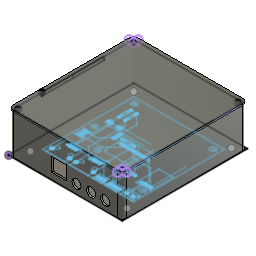
krabice - štít v2 (Autodesk Fusion 360 design; units mm, degrees)
Autodesk Fusion 360 part; units mm, degrees
note: some values were not read from the file. Set by a fixed rule: which sketch regions a step uses.
sketch "Base" plane through (0, 0, 0) normal (0, 1, 0) x (1, 0, 0) in component "Top"
  line L0 (0, 0) -> (100, 0)
  line L1 (100, 0) -> (100, 110)
  line L2 (100, 110) -> (0, 110)
  line L3 (0, 110) -> (0, 0)
  dimension "d6" = 100
  dimension "d7" = 110
  constraint horizontal L0
  constraint vertical L1
  constraint horizontal L2
  constraint vertical L3
  constraint coincident L0.start L3.end
  measures "d6" distance of L0.start L0.end
  measures "d7" distance of L0.start L2.end
extrude "Extrude1" add sketch "Base" along normal blind 35 makes body 1 in component "Top"
fillet "Fillet1" radius 4 4 edges at (100, 17.5, 0) (0, 17.5, 0) (100, 17.5, -110) (0, 17.5, -110) on bodies 1 in component "Top"
shell "Shell1" thickness 1.5 removed faces 1 at (33.3333, 35, -72) on bodies 1 in component "Top"
sketch "Knob" plane through (1.5, 0, 0) normal (1, 0, 0) x (0, 0, -1) in component "Top"
  line L0 (106, 1.5) -> (106, 35)
  line L1 (106, 35) -> (4, 35)
  line L2 (4, 35) -> (4, 1.5)
  line L3 (4, 1.5) -> (106, 1.5)
  line L4 (27.5, 35) -> (82.5, 35)
  line L5 (82.5, 35) -> (82.5, 32)
  line L6 (82.5, 32) -> (27.5, 32)
  line L7 (27.5, 32) -> (27.5, 35)
  line L8 (55, 35) -> (55, 32) construction
  dimension "d12" = 55
  dimension "d13" = 3
  constraint horizontal L4
  constraint vertical L5
  constraint horizontal L6
  constraint vertical L7
  constraint coincident L1 L4.start
  constraint midpoint L1 L8.start
  constraint midpoint L6 L8.end
  constraint vertical L8
  measures "d12" distance of L5.end L6.end
  measures "d13" distance of L4.end L5.end
extrude "Extrude2" add sketch "Knob" along normal blind 6 draft -45 contours L1 L4 L5 L6 L7 bodies 1 in component "Top"
ref_plane "WorkPlane2" through (50, 17.5, -55) normal (-1, 0, 0) x (0, 0, 1) in component "Top"
mirror "Mirror1" about plane through (50, 17.5, -55) normal (-1, 0, 0) of "Extrude2" in component "Top"
sketch "Top" plane through (0, 35, 0) normal (0, 1, 0) x (-1, 0, 0) in component "Base"
  line L0 (-100, -4) -> (-100, -106)
  arc A0 (-100, -106) -> (-96, -110) centre (-96, -106) ccw
  line L1 (-96, -110) -> (-4, -110)
  arc A1 (-4, -110) -> (0, -106) centre (-4, -106) ccw
  line L2 (0, -106) -> (0, -4)
  arc A2 (0, -4) -> (-4, 0) centre (-4, -4) ccw
  line L3 (-4, 0) -> (-96, 0)
  arc A3 (-96, 0) -> (-100, -4) centre (-96, -4) ccw
  arc A4 (-96, -1.5) -> (-98.5, -4) centre (-96, -4) ccw
  line L4 (-96, -1.5) -> (-4, -1.5)
  arc A5 (-1.5, -4) -> (-4, -1.5) centre (-4, -4) ccw
  line L5 (-1.5, -27.5) -> (-1.5, -82.5)
  arc A6 (-4, -108.5) -> (-1.5, -106) centre (-4, -106) ccw
  line L6 (-4, -108.5) -> (-96, -108.5)
  arc A7 (-98.5, -106) -> (-96, -108.5) centre (-96, -106) ccw
  line L7 (-98.5, -82.5) -> (-98.5, -27.5)
  line L8 (-98.5, -27.5) -> (-98.5, -4)
  line L9 (-1.5, -4) -> (-1.5, -27.5)
  line L10 (-1.5, -82.5) -> (-1.5, -106)
  line L11 (-98.5, -106) -> (-98.5, -82.5)
extrude "Extrude1'" add sketch "Top" along normal blind 1.5 separate body contours L0 A0 L1 A1 L2 A2 L3 A3 | A4 L4 A5 L5 A6 L6 A7 L7 L8 L9 L10 L11 makes body 2 in component "Base"
sketch "Lip" plane through (0, 35, 0) normal (0, -1, 0) x (1, 0, 0) in component "Base"
  arc A0 (100, -4) -> (96, 0) centre (96, -4) ccw
  line L0 (96, 0) -> (4, 0)
  arc A1 (4, 0) -> (0, -4) centre (4, -4) ccw
  line L1 (0, -4) -> (0, -106)
  arc A2 (0, -106) -> (4, -110) centre (4, -106) ccw
  line L2 (4, -110) -> (96, -110)
  arc A3 (96, -110) -> (100, -106) centre (96, -106) ccw
  line L3 (100, -106) -> (100, -4)
  line L4 (98.3, -106) -> (98.3, -4)
  arc A4 (98.3, -4) -> (96, -1.7) centre (96, -4) ccw
  line L5 (96, -1.7) -> (4, -1.7)
  arc A5 (4, -1.7) -> (1.7, -4) centre (4, -4) ccw
  line L6 (1.7, -4) -> (1.7, -106)
  arc A6 (1.7, -106) -> (4, -108.3) centre (4, -106) ccw
  line L7 (4, -108.3) -> (96, -108.3)
  arc A7 (96, -108.3) -> (98.3, -106) centre (96, -106) ccw
  dimension "d19" = 1.7
extrude "Extrude2'" add sketch "Lip" along normal blind 3 contours L4 A4 L5 A5 L6 A6 L7 A7 bodies 2 in component "Base"
extrude "Extrude3" cut sketch "Knob" along normal blind 3 draft -45 from surface at 0.2 contours L1 L4 L5 L6 L7 bodies 2 in component "Base"
mirror "Mirror1'" about plane through (50, 17.5, -55) normal (-1, 0, 0) of "Extrude3" in component "Base"
shell "Shell1'" thickness 1.5 removed faces 1 at (66.1, 32, -64.1667) on bodies 2 in component "Base"
chamfer "Chamfer1" distance 0.6 angle 45 2 edges at (1.7, 32, -55) (98.3, 32, -55) on bodies 2 in component "Base"
sketch "PCB Mount" plane through (0, 35, 0) normal (0, -1, 0) x (1, 0, 0) in component "Base"
  arc A0 (100, -4) -> (96, 0) centre (96, -4) ccw construction
  arc A1 (0, -106) -> (4, -110) centre (4, -106) ccw construction
sketch "PCB_Slave_2021-08-24" plane through (0, 1.5, -25) normal (0, 1, 0) x (1, 0, 0)
  line L0 (57.578, 9.4539) -> (57.578, 31.463)
  line L1 (85.899, 11.27) -> (84.5401, 12.6289)
  line L2 (84.5401, 12.6289) -> (82.7926, 12.6289)
  line L3 (30.3848, 47.0992) -> (30.3848, 43.147)
  line L4 (34.6494, 52.9946) -> (34.6494, 38.194)
  line L5 (51.482, 37.559) -> (57.578, 31.463)
  line L6 (49.958, 35.4) -> (49.958, 31.463)
  line L7 (43.9915, 8.4836) -> (50.245, 8.4836)
  line L8 (30.3848, 14.9276) -> (39.6304, 5.682)
  line L9 (20.875, 44.4018) -> (21.9215, 44.4018)
  line L10 (21.9215, 44.4018) -> (22.968, 43.3553)
  line L11 (62.465, -3.7363) -> (64.0169, -5.2857)
  line L12 (88.439, 42.131) -> (88.439, 11.27)
  line L13 (21.698, 9.1212) -> (21.698, 18.697)
  line L14 (30.3848, 43.147) -> (30.3848, 14.9276)
  line L15 (26.082, 61.562) -> (34.6494, 52.9946)
  line L16 (72.437, 13.683) -> (65.198, 20.922)
  line L17 (26.082, 51.402) -> (30.3848, 47.0992)
  line L18 (60.118, 9.4539) -> (73.3057, -3.7363)
  line L19 (64.0169, -5.2857) -> (74.2963, -5.2857)
  line L20 (65.198, 20.922) -> (65.198, 31.463)
  line L21 (70.7657, -3.7363) -> (57.578, 9.4539)
  line L22 (74.2963, -5.2857) -> (75.8457, -3.7363)
  line L23 (61.5582, 14.4018) -> (62.277, 13.683)
  line L24 (60.118, 31.463) -> (60.118, 9.4539)
  line L25 (59.102, 32.479) -> (60.118, 31.463)
  line L26 (39.6304, 5.682) -> (43.7299, 5.682)
  line L27 (43.7299, 5.682) -> (45.2615, 7.2136)
  line L28 (87.6364, -3.335) -> (83.359, 0.9424)
  line L29 (20.875, 51.402) -> (20.875, 44.4018)
  line L30 (82.0687, -2.7686) -> (82.6376, -3.335)
  line L31 (22.968, 43.3553) -> (22.968, 9.7536)
  line L32 (66.8033, 35.6083) -> (64.8373, 33.6423)
  line L33 (64.8373, 33.6423) -> (82.7926, 15.6871)
  line L34 (61.5582, 41.0718) -> (61.5582, 14.4018)
  line L35 (17.3139, 23.081) -> (21.6218, 27.3888)
  line L36 (50.245, 8.4836) -> (62.465, -3.7363)
  line L37 (24.238, 7.2136) -> (23.603, 7.2136)
  line L38 (83.359, 0.9424) -> (83.359, 11.27)
  line L39 (43.9915, 8.4836) -> (42.7215, 7.2136)
  line L40 (49.958, 13.1801) -> (49.958, 31.463)
  line L41 (23.603, 7.2136) -> (21.698, 9.1212)
  line L42 (82.7926, 15.6871) -> (82.7926, 12.6289)
  line L43 (43.9915, 9.7536) -> (43.9915, 8.4836)
  line L44 (82.7926, 12.6289) -> (82.0687, 11.905)
  line L45 (64.8373, 33.6423) -> (62.658, 31.463)
  line L46 (21.6218, 27.3888) -> (21.6218, 43.147)
  line L47 (21.698, 18.697) -> (17.3139, 23.081)
  line L48 (49.704, 35.654) -> (49.958, 35.4)
  line L49 (46.5315, 9.7536) -> (49.958, 13.1801)
  line L50 (20.875, 44.4018) -> (19.6202, 43.147)
  line L51 (82.0687, 11.905) -> (82.0687, -2.7686)
  line L52 (92, 73) -> (92, -7)
  line L53 (12, 73) -> (92, 73)
  line L54 (12, -7) -> (12, 73)
  line L55 (92, -7) -> (12, -7)
  line L56 (66.6763, -5.2857) -> (68.2257, -3.7363)
  line L57 (57.385, -3.7363) -> (58.9369, -5.2857)
  line L58 (36.496, 20.541) -> (17.3139, 20.541)
  line L59 (65.198, 38.194) -> (34.6494, 38.194)
  line L60 (41.5227, 8.415) -> (25.4394, 8.415)
  line L61 (68.2257, 9.4717) -> (72.437, 13.683)
  line L62 (53.768, 31.0007) -> (53.768, 32.0472)
  line L63 (73.707, 26.002) -> (58.7667, 26.002)
  line L64 (42.7215, 7.2136) -> (41.5227, 8.415)
  line L65 (82.6376, -3.335) -> (76.247, -3.335)
  line L66 (47.418, 31.463) -> (36.496, 20.541)
  line L67 (52.7012, 33.114) -> (34.6494, 33.114)
  line L68 (22.5412, 40.226) -> (19.6202, 43.147)
  line L69 (26.082, 61.562) -> (20.875, 61.562)
  line L70 (31.4008, 44.163) -> (30.3848, 43.147)
  line L71 (65.198, 42.004) -> (65.198, 38.194)
  line L72 (76.247, -3.335) -> (75.8457, -3.7363)
  line L73 (58.7667, 26.002) -> (53.768, 31.0007)
  line L74 (88.439, 11.27) -> (73.707, 26.002)
  line L75 (59.925, -3.7363) -> (62.277, -1.3843)
  line L76 (68.2257, -3.7363) -> (68.2257, 9.4717)
  line L77 (25.4394, 8.415) -> (24.238, 7.2136)
  line L78 (55.927, 44.163) -> (31.4008, 44.163)
  line L79 (17.3139, 25.621) -> (27.1564, 25.621)
  line L80 (62.277, -1.3843) -> (62.277, 13.683)
  line L81 (39.544, 35.654) -> (34.6494, 35.654)
  line L82 (53.26, 40.226) -> (22.5412, 40.226)
  line L83 (28.3832, 43.147) -> (21.6218, 43.147)
  line L84 (27.1564, 25.621) -> (34.6494, 33.114)
  line L85 (65.198, 38.194) -> (65.198, 31.463)
  line L86 (58.9369, -5.2857) -> (66.6763, -5.2857)
  line L87 (53.768, 32.0472) -> (52.7012, 33.114)
  line L88 (64.817, 14.699) -> (69.897, 14.699)
  line L89 (63.9349, -0.735) -> (63.9349, -7.035)
  line L90 (55.9149, -0.735) -> (55.9149, -7.035)
  line L91 (55.9149, -7.035) -> (63.9349, -7.035)
  line L92 (33.3794, 31.844) -> (33.3794, 39.464)
  line L93 (55.9149, -0.735) -> (63.9349, -0.735)
  line L94 (33.3794, 39.464) -> (35.9194, 39.464)
  line L95 (64.817, 12.667) -> (64.817, 14.699)
  line L96 (66.756, -0.735) -> (77.316, -0.735)
  line L97 (30.384, 41.147) -> (30.384, 42.163)
  line L98 (69.897, 13.683) -> (72.437, 13.683)
  line L99 (35.9194, 39.464) -> (35.9194, 31.844)
  line L100 (20.3141, 27.091) -> (14.0141, 27.091)
  line L101 (66.756, -0.735) -> (66.756, -7.035)
  line L102 (66.756, -2.277) -> (77.316, -2.277)
  line L103 (55.9149, -2.277) -> (63.9349, -2.277)
  line L104 (20.3141, 27.091) -> (20.3141, 19.071)
  line L105 (15.7524, 27.091) -> (15.7524, 19.071)
  line L106 (66.756, -6.5047) -> (77.316, -6.5047)
  line L107 (78.2789, 21.43) -> (78.2789, 29.05)
  line L108 (79.5489, 10.3708) -> (79.5489, 10)
  line L109 (65.7314, 18.7376) -> (41.83, 18.763)
  line L110 (62.277, 13.683) -> (64.817, 13.683)
  line L111 (19.1049, 44.6469) -> (20.1209, 44.6469)
  line L112 (79.5489, 10) -> (89.7089, 10)
  line L113 (20.3141, 19.071) -> (14.0141, 19.071)
  line L114 (66.756, -5.2967) -> (77.316, -5.2967)
  line L115 (79.5489, 12.54) -> (79.5489, 10.3708)
  line L116 (69.897, 14.699) -> (69.897, 12.667)
  line L117 (39.798, 20.7188) -> (39.798, 30.701)
  line L118 (14.0141, 27.091) -> (14.0141, 19.071)
  line L119 (21.891, 53.942) -> (19.859, 53.942)
  line L120 (19.859, 53.942) -> (19.859, 59.022)
  line L121 (69.897, 12.667) -> (64.817, 12.667)
  line L122 (41.83, 32.733) -> (65.7314, 32.733)
  line L123 (66.756, -7.035) -> (77.316, -7.035)
  line L124 (90.8519, 29.05) -> (90.8519, 8.73)
  line L125 (19.621, 45.147) -> (19.621, 44.131)
  line L126 (19.859, 59.022) -> (21.891, 59.022)
  line L127 (27.098, 59.022) -> (27.098, 53.942)
  line L128 (55.9149, -5.2967) -> (63.9349, -5.2967)
  line L129 (25.066, 59.022) -> (27.098, 59.022)
  line L130 (42.084, 36.67) -> (47.164, 36.67)
  line L131 (47.164, 35.654) -> (49.704, 35.654)
  line L132 (80.137, 0.665) -> (90.137, 0.665)
  line L133 (47.164, 36.67) -> (47.164, 34.638)
  line L134 (80.137, 0.665) -> (80.137, -7.035)
  line L135 (35.9194, 31.844) -> (33.3794, 31.844)
  line L136 (89.7089, 12.54) -> (79.5489, 12.54)
  line L137 (20.875, 53.942) -> (20.875, 51.402)
  line L138 (55.9149, -6.5047) -> (63.9349, -6.5047)
  line L139 (78.2789, 8.73) -> (78.2789, 21.43)
  line L140 (30.9001, 41.6471) -> (29.8841, 41.6471)
  line L141 (26.082, 53.942) -> (26.082, 51.402)
  line L142 (27.098, 53.942) -> (25.066, 53.942)
  line L143 (47.164, 34.638) -> (42.084, 34.638)
  line L144 (18.772, 27.091) -> (18.772, 19.071)
  line L145 (77.316, -0.735) -> (77.316, -7.035)
  line L146 (67.738, 30.7264) -> (67.738, 20.7442)
  line L147 (25.066, 53.942) -> (25.066, 59.022)
  line L148 (90.8519, 8.73) -> (78.2789, 8.73)
  line L149 (90.137, 0.665) -> (90.137, -7.035)
  line L150 (42.084, 34.638) -> (42.084, 36.67)
  line L151 (80.137, -7.035) -> (90.137, -7.035)
  line L152 (20.875, 61.562) -> (20.875, 59.022)
  line L153 (21.891, 59.022) -> (21.891, 53.942)
  line L154 (14.5444, 27.091) -> (14.5444, 19.071)
  line L155 (39.544, 35.654) -> (42.084, 35.654)
  line L156 (26.082, 61.562) -> (26.082, 59.022)
  line L157 (89.7089, 10) -> (89.7089, 12.54)
  line L158 (78.2789, 29.05) -> (90.8519, 29.05)
  line L159 (36.0522, 11.365) -> (51.9323, 11.365)
  arc A0 (65.739, 18.733) -> (67.738, 20.733) centre (65.739, 20.732) ccw
  line L160 (51.9323, -7.035) -> (36.0522, -7.035)
  arc A1 (39.83, 20.763) -> (41.829, 18.763) centre (41.829, 20.762) ccw
  line L161 (90.845, -1.7086) -> (90.217, -1.7086)
  arc A2 (67.738, 30.733) -> (65.739, 32.733) centre (65.739, 30.734) ccw
  line L162 (15.0279, 11.365) -> (30.908, 11.365)
  line L163 (80.137, -5.1796) -> (90.137, -5.1796)
  circle A3 centre (20.621, 43.147) radius 2.5001
  line L164 (80.137, -1.1344) -> (90.137, -1.1344)
  line L165 (30.908, 11.365) -> (30.908, -7.035)
  line L166 (51.9323, 11.365) -> (51.9323, -7.035)
  line L167 (36.0522, -7.035) -> (36.0522, 11.365)
  line L168 (30.908, -7.035) -> (15.0279, -7.035)
  line L169 (15.0279, -7.035) -> (15.0279, 11.365)
  circle A4 centre (29.384, 43.147) radius 2.5001
  arc A5 (41.797, 32.701) -> (39.798, 30.701) centre (41.797, 30.702) ccw
  line L170 (90.845, -0.668) -> (90.845, -1.7086)
  line L171 (90.217, -0.668) -> (90.845, -0.668)
  line L172 (69.897, 13.683) -> (72.437, 13.683)
  line L173 (42.084, 34.638) -> (42.084, 36.67)
  line L174 (64.817, 12.667) -> (64.817, 14.699)
  line L175 (27.098, 59.022) -> (27.098, 53.942)
  line L176 (20.875, 61.562) -> (20.875, 59.022)
  line L177 (25.066, 53.942) -> (25.066, 59.022)
  line L178 (47.164, 36.67) -> (47.164, 34.638)
  line L179 (26.082, 53.942) -> (26.082, 51.402)
  line L180 (27.098, 53.942) -> (25.066, 53.942)
  line L181 (69.897, 12.667) -> (64.817, 12.667)
  line L182 (21.891, 59.022) -> (21.891, 53.942)
  line L183 (42.084, 36.67) -> (47.164, 36.67)
  line L184 (21.891, 53.942) -> (19.859, 53.942)
  line L185 (39.544, 35.654) -> (42.084, 35.654)
  line L186 (69.897, 14.699) -> (69.897, 12.667)
  line L187 (19.859, 53.942) -> (19.859, 59.022)
  line L188 (47.164, 35.654) -> (49.704, 35.654)
  line L189 (26.082, 61.562) -> (26.082, 59.022)
  line L190 (62.277, 13.683) -> (64.817, 13.683)
  line L191 (25.066, 59.022) -> (27.098, 59.022)
  line L192 (47.164, 34.638) -> (42.084, 34.638)
  line L193 (19.859, 59.022) -> (21.891, 59.022)
  line L194 (20.875, 53.942) -> (20.875, 51.402)
  line L195 (64.817, 14.699) -> (69.897, 14.699)
  circle A6 centre (47.8023, 7.2149) radius 0.8008
  circle A7 centre (15.2179, -2.1399) radius 1.3008
  circle A8 centre (42.7223, 7.215) radius 0.4805
  circle A9 centre (51.7423, -2.14) radius 0.8325
  circle A10 centre (46.5323, 9.755) radius 0.4805
  circle A11 centre (41.4523, 9.755) radius 0.4805
  circle A12 centre (45.2623, 7.215) radius 0.4805
  circle A13 centre (87.6371, -3.335) radius 1.1254
  circle A14 centre (51.7423, -2.1399) radius 1.3008
  circle A15 centre (28.048, 9.755) radius 0.4805
  circle A16 centre (41.4523, 9.7549) radius 0.8008
  circle A17 centre (42.7223, 7.2149) radius 0.8008
  circle A18 centre (22.968, 9.755) radius 0.4805
  circle A19 centre (46.5323, 9.7549) radius 0.8008
  circle A20 centre (20.428, 9.7549) radius 0.8008
  circle A21 centre (49.0723, 9.755) radius 0.4805
  circle A22 centre (36.2423, -2.14) radius 0.8325
  circle A23 centre (43.9923, 9.755) radius 0.4805
  circle A24 centre (22.968, 9.7549) radius 0.8008
  circle A25 centre (28.048, 9.7549) radius 0.8008
  circle A26 centre (15.218, -2.14) radius 0.8325
  circle A27 centre (80.819, 11.27) radius 0.5317
  circle A28 centre (82.637, -3.335) radius 0.7162
  circle A29 centre (45.2623, 7.2149) radius 0.8008
  circle A30 centre (25.508, 9.755) radius 0.4805
  circle A31 centre (36.2423, -2.1399) radius 1.3008
  circle A32 centre (47.8023, 7.215) radius 0.4805
  circle A33 centre (43.9923, 9.7549) radius 0.8008
  circle A34 centre (40.1823, 7.2149) radius 0.4805
  circle A35 centre (19.158, 7.2149) radius 0.4805
  circle A36 centre (25.508, 9.7549) radius 0.8008
  circle A37 centre (49.0723, 9.7549) radius 0.8008
  circle A38 centre (24.238, 7.215) radius 0.4805
  circle A39 centre (34.6494, 38.194) radius 0.9008
  circle A40 centre (34.6494, 33.114) radius 0.9008
  circle A41 centre (34.6494, 35.654) radius 0.9008
  circle A42 centre (57.578, 31.463) radius 0.4877
  circle A43 centre (57.578, 31.463) radius 0.8128
  circle A44 centre (65.198, 31.463) radius 0.4877
  circle A45 centre (17.3141, 20.541) radius 0.6665
  circle A46 centre (65.198, 31.463) radius 0.8128
  circle A47 centre (17.3142, 25.621) radius 1.0254
  circle A48 centre (17.3141, 25.621) radius 0.6665
  circle A49 centre (62.658, 31.463) radius 0.4877
  circle A50 centre (34.6494, 33.114) radius 0.5829
  circle A51 centre (34.6494, 38.194) radius 0.5829
  circle A52 centre (34.6494, 35.654) radius 0.5829
  circle A53 centre (73.3059, -3.7351) radius 1.0254
  circle A54 centre (68.2259, -3.7351) radius 1.0254
  circle A55 centre (20.875, 61.562) radius 0.4875
  circle A56 centre (44.878, 31.463) radius 0.4877
  circle A57 centre (21.621, 43.147) radius 0.4156
  circle A58 centre (55.038, 31.463) radius 0.4877
  circle A59 centre (17.3142, 23.081) radius 1.0254
  circle A60 centre (62.277, 13.683) radius 0.8128
  circle A61 centre (52.498, 31.463) radius 0.4877
  circle A62 centre (62.658, 31.463) radius 0.8128
  circle A63 centre (59.925, -3.7351) radius 1.0254
  circle A64 centre (57.3849, -3.735) radius 0.6665
  circle A65 centre (85.899, 11.27) radius 0.8508
  circle A66 centre (83.359, 11.27) radius 0.8508
  circle A67 centre (17.3142, 20.541) radius 1.0254
  circle A68 centre (19.621, 43.147) radius 0.6754
  circle A69 centre (55.038, 31.463) radius 0.8128
  circle A70 centre (72.437, 13.683) radius 0.8128
  circle A71 centre (59.9249, -3.735) radius 0.6665
  circle A72 centre (57.385, -3.7351) radius 1.0254
  circle A73 centre (21.621, 43.147) radius 0.6754
  circle A74 centre (42.338, 31.463) radius 0.8128
  circle A75 centre (70.766, -3.735) radius 0.6665
  circle A76 centre (83.359, 11.27) radius 0.5317
  circle A77 centre (88.439, 11.27) radius 0.5317
  circle A78 centre (20.875, 51.402) radius 0.8128
  circle A79 centre (49.958, 31.463) radius 0.4877
  circle A80 centre (62.465, -3.7351) radius 1.0254
  circle A81 centre (73.306, -3.735) radius 0.6665
  circle A82 centre (88.439, 11.27) radius 0.8508
  circle A83 centre (19.621, 43.147) radius 0.4156
  circle A84 centre (26.082, 51.402) radius 0.8128
  circle A85 centre (26.082, 61.562) radius 0.8128
  circle A86 centre (42.338, 31.463) radius 0.4877
  circle A87 centre (85.899, 11.27) radius 0.5317
  circle A88 centre (26.082, 61.562) radius 0.4875
  circle A89 centre (26.082, 51.402) radius 0.4875
  circle A90 centre (60.118, 31.463) radius 0.8128
  circle A91 centre (68.226, -3.735) radius 0.6665
  circle A92 centre (20.875, 61.562) radius 0.8128
  circle A93 centre (62.277, 13.683) radius 0.4875
  circle A94 centre (49.704, 35.654) radius 0.4875
  circle A95 centre (49.704, 35.654) radius 0.8128
  circle A96 centre (47.418, 31.463) radius 0.8128
  circle A97 centre (28.384, 43.147) radius 0.4156
  circle A98 centre (17.3141, 23.081) radius 0.6665
  circle A99 centre (60.118, 31.463) radius 0.4877
  circle A100 centre (28.384, 43.147) radius 0.6754
  circle A101 centre (49.958, 31.463) radius 0.8128
  circle A102 centre (62.4649, -3.735) radius 0.6665
  circle A103 centre (30.384, 43.147) radius 0.6754
  circle A104 centre (75.8459, -3.7351) radius 1.0254
  circle A105 centre (21.698, 7.2149) radius 0.8008
  circle A106 centre (44.878, 31.463) radius 0.8128
  circle A107 centre (75.846, -3.735) radius 0.6665
  circle A108 centre (20.428, 9.755) radius 0.4805
  circle A109 centre (70.7659, -3.7351) radius 1.0254
  circle A110 centre (72.437, 13.683) radius 0.4875
  circle A111 centre (52.498, 31.463) radius 0.8128
  circle A112 centre (20.875, 51.402) radius 0.4875
  circle A113 centre (30.384, 43.147) radius 0.4156
  circle A114 centre (39.544, 35.654) radius 0.8128
  circle A115 centre (39.544, 35.654) radius 0.4875
  circle A116 centre (47.418, 31.463) radius 0.4877
  circle A117 centre (30.718, -2.1399) radius 1.3008
  circle A118 centre (82.6371, -3.335) radius 1.1254
  circle A119 centre (26.778, 7.215) radius 0.4805
  circle A120 centre (24.238, 7.2149) radius 0.8008
  circle A121 centre (21.698, 7.215) radius 0.4805
  circle A122 centre (30.718, -2.14) radius 0.8325
  circle A123 centre (26.778, 7.2149) radius 0.8008
  circle A124 centre (87.637, -3.335) radius 0.7162
  circle A125 centre (52.498, 31.463) radius 0.8128
  circle A126 centre (44.878, 31.463) radius 0.4877
  circle A127 centre (20.875, 51.402) radius 0.8128
  circle A128 centre (17.3141, 23.081) radius 0.6665
  circle A129 centre (57.3849, -3.735) radius 0.6665
  circle A130 centre (72.437, 13.683) radius 0.8128
  circle A131 centre (57.578, 31.463) radius 0.8128
  circle A132 centre (62.277, 13.683) radius 0.4875
  circle A133 centre (17.3142, 20.541) radius 1.0254
  circle A134 centre (34.6494, 33.114) radius 0.5829
  circle A135 centre (21.621, 43.147) radius 0.6754
  circle A136 centre (34.6494, 33.114) radius 0.9008
  circle A137 centre (34.6494, 38.194) radius 0.5829
  circle A138 centre (70.766, -3.735) radius 0.6665
  circle A139 centre (57.578, 31.463) radius 0.4877
  circle A140 centre (47.418, 31.463) radius 0.4877
  circle A141 centre (17.3141, 20.541) radius 0.6665
  circle A142 centre (49.958, 31.463) radius 0.8128
  circle A143 centre (83.359, 11.27) radius 0.8508
  circle A144 centre (75.8459, -3.7351) radius 1.0254
  circle A145 centre (75.846, -3.735) radius 0.6665
  circle A146 centre (60.118, 31.463) radius 0.8128
  circle A147 centre (85.899, 11.27) radius 0.5317
  circle A148 centre (19.621, 43.147) radius 0.6754
  circle A149 centre (83.359, 11.27) radius 0.5317
  circle A150 centre (59.925, -3.7351) radius 1.0254
  circle A151 centre (17.3142, 23.081) radius 1.0254
  circle A152 centre (62.277, 13.683) radius 0.8128
  circle A153 centre (73.306, -3.735) radius 0.6665
  circle A154 centre (20.875, 51.402) radius 0.4875
  circle A155 centre (52.498, 31.463) radius 0.4877
  circle A156 centre (34.6494, 35.654) radius 0.5829
  circle A157 centre (47.418, 31.463) radius 0.8128
  circle A158 centre (65.198, 31.463) radius 0.4877
  circle A159 centre (55.038, 31.463) radius 0.4877
  circle A160 centre (62.4649, -3.735) radius 0.6665
  circle A161 centre (62.465, -3.7351) radius 1.0254
  circle A162 centre (34.6494, 35.654) radius 0.9008
  circle A163 centre (88.439, 11.27) radius 0.8508
  circle A164 centre (44.878, 31.463) radius 0.8128
  circle A165 centre (49.958, 31.463) radius 0.4877
  circle A166 centre (73.3059, -3.7351) radius 1.0254
  circle A167 centre (85.899, 11.27) radius 0.8508
  circle A168 centre (62.658, 31.463) radius 0.4877
  circle A169 centre (42.338, 31.463) radius 0.8128
  circle A170 centre (34.6494, 38.194) radius 0.9008
  circle A171 centre (65.198, 31.463) radius 0.8128
  circle A172 centre (59.9249, -3.735) radius 0.6665
  circle A173 centre (17.3142, 25.621) radius 1.0254
  circle A174 centre (21.621, 43.147) radius 0.4156
  circle A175 centre (28.384, 43.147) radius 0.6754
  circle A176 centre (20.875, 61.562) radius 0.8128
  circle A177 centre (55.038, 31.463) radius 0.8128
  circle A178 centre (72.437, 13.683) radius 0.4875
  circle A179 centre (42.338, 31.463) radius 0.4877
  circle A180 centre (68.2259, -3.7351) radius 1.0254
  circle A181 centre (57.385, -3.7351) radius 1.0254
  circle A182 centre (17.3141, 25.621) radius 0.6665
  circle A183 centre (60.118, 31.463) radius 0.4877
  circle A184 centre (19.621, 43.147) radius 0.4156
  circle A185 centre (88.439, 11.27) radius 0.5317
  circle A186 centre (70.7659, -3.7351) radius 1.0254
  circle A187 centre (68.226, -3.735) radius 0.6665
  circle A188 centre (62.658, 31.463) radius 0.8128
  circle A189 centre (25.508, 9.755) radius 0.4805
  circle A190 centre (20.428, 9.755) radius 0.4805
  circle A191 centre (46.5323, 9.755) radius 0.4805
  circle A192 centre (45.2623, 7.215) radius 0.4805
  circle A193 centre (41.4523, 9.755) radius 0.4805
  circle A194 centre (87.637, -3.335) radius 0.7162
  circle A195 centre (43.9923, 9.755) radius 0.4805
  circle A196 centre (41.4523, 9.7549) radius 0.8008
  circle A197 centre (47.8023, 7.2149) radius 0.8008
  circle A198 centre (28.048, 9.755) radius 0.4805
  circle A199 centre (26.082, 61.562) radius 0.8128
  circle A200 centre (28.384, 43.147) radius 0.4156
  circle A201 centre (45.2623, 7.2149) radius 0.8008
  circle A202 centre (42.7223, 7.215) radius 0.4805
  circle A203 centre (28.048, 9.7549) radius 0.8008
  circle A204 centre (15.2179, -2.1399) radius 1.3008
  circle A205 centre (43.9923, 9.7549) radius 0.8008
  circle A206 centre (39.544, 35.654) radius 0.8128
  circle A207 centre (42.7223, 7.2149) radius 0.8008
  circle A208 centre (20.875, 61.562) radius 0.4875
  circle A209 centre (49.0723, 9.7549) radius 0.8008
  circle A210 centre (26.082, 51.402) radius 0.8128
  circle A211 centre (24.238, 7.2149) radius 0.8008
  circle A212 centre (22.968, 9.7549) radius 0.8008
  circle A213 centre (36.2423, -2.14) radius 0.8325
  circle A214 centre (51.7423, -2.1399) radius 1.3008
  circle A215 centre (30.718, -2.1399) radius 1.3008
  circle A216 centre (30.384, 43.147) radius 0.6754
  circle A217 centre (21.698, 7.215) radius 0.4805
  circle A218 centre (82.637, -3.335) radius 0.7162
  circle A219 centre (47.8023, 7.215) radius 0.4805
  circle A220 centre (36.2423, -2.1399) radius 1.3008
  circle A221 centre (26.082, 51.402) radius 0.4875
  circle A222 centre (30.718, -2.14) radius 0.8325
  circle A223 centre (87.6371, -3.335) radius 1.1254
  circle A224 centre (21.698, 7.2149) radius 0.8008
  circle A225 centre (26.778, 7.215) radius 0.4805
  circle A226 centre (26.778, 7.2149) radius 0.8008
  circle A227 centre (25.508, 9.7549) radius 0.8008
  circle A228 centre (49.0723, 9.755) radius 0.4805
  circle A229 centre (82.6371, -3.335) radius 1.1254
  circle A230 centre (20.428, 9.7549) radius 0.8008
  circle A231 centre (30.384, 43.147) radius 0.4156
  circle A232 centre (24.238, 7.215) radius 0.4805
  circle A233 centre (49.704, 35.654) radius 0.4875
  circle A234 centre (15.218, -2.14) radius 0.8325
  circle A235 centre (22.968, 9.755) radius 0.4805
  circle A236 centre (51.7423, -2.14) radius 0.8325
  circle A237 centre (49.704, 35.654) radius 0.8128
  circle A238 centre (46.5323, 9.7549) radius 0.8008
  circle A239 centre (39.544, 35.654) radius 0.4875
  circle A240 centre (26.082, 61.562) radius 0.4875
  circle A241 centre (19.158, 7.2149) radius 0.4805
  circle A242 centre (40.1823, 7.2149) radius 0.4805
  circle A243 centre (80.819, 11.27) radius 0.5317
  circle A244 centre (34.6494, 35.654) radius 0.55
  circle A245 centre (34.6494, 35.654) radius 0.85
  circle A246 centre (34.6494, 33.114) radius 0.55
  circle A247 centre (60.118, 31.463) radius 0.4572
  circle A248 centre (62.658, 31.463) radius 0.762
  circle A249 centre (62.658, 31.463) radius 0.4572
  circle A250 centre (34.6494, 38.194) radius 0.55
  circle A251 centre (17.3141, 25.621) radius 0.65
  circle A252 centre (34.6494, 33.114) radius 0.85
  circle A253 centre (17.3142, 23.081) radius 1
  circle A254 centre (17.3141, 20.541) radius 0.65
  circle A255 centre (65.198, 31.463) radius 0.762
  circle A256 centre (49.958, 31.463) radius 0.762
  circle A257 centre (57.578, 31.463) radius 0.762
  circle A258 centre (68.2259, -3.7351) radius 1
  circle A259 centre (20.875, 51.402) radius 0.457
  circle A260 centre (55.038, 31.463) radius 0.4572
  circle A261 centre (68.226, -3.735) radius 0.65
  circle A262 centre (60.118, 31.463) radius 0.762
  circle A263 centre (57.578, 31.463) radius 0.4572
  circle A264 centre (44.878, 31.463) radius 0.4572
  circle A265 centre (72.437, 13.683) radius 0.762
  circle A266 centre (20.875, 51.402) radius 0.762
  circle A267 centre (62.277, 13.683) radius 0.457
  circle A268 centre (62.4649, -3.735) radius 0.65
  circle A269 centre (70.7659, -3.7351) radius 1
  circle A270 centre (17.3141, 23.081) radius 0.65
  circle A271 centre (55.038, 31.463) radius 0.762
  circle A272 centre (42.338, 31.463) radius 0.4572
  circle A273 centre (62.277, 13.683) radius 0.762
  circle A274 centre (21.621, 43.147) radius 0.65
  circle A275 centre (17.3142, 25.621) radius 1
  circle A276 centre (52.498, 31.463) radius 0.4572
  circle A277 centre (57.385, -3.7351) radius 1
  circle A278 centre (19.621, 43.147) radius 0.65
  circle A279 centre (19.621, 43.147) radius 0.4
  circle A280 centre (72.437, 13.683) radius 0.457
  circle A281 centre (47.418, 31.463) radius 0.4572
  circle A282 centre (49.958, 31.463) radius 0.4572
  circle A283 centre (88.439, 11.27) radius 0.5
  circle A284 centre (88.439, 11.27) radius 0.8
  circle A285 centre (75.8459, -3.7351) radius 1
  circle A286 centre (17.3142, 20.541) radius 1
  circle A287 centre (21.621, 43.147) radius 0.4
  circle A288 centre (39.544, 35.654) radius 0.457
  circle A289 centre (20.875, 61.562) radius 0.762
  circle A290 centre (44.878, 31.463) radius 0.762
  circle A291 centre (26.082, 61.562) radius 0.457
  circle A292 centre (42.338, 31.463) radius 0.762
  circle A293 centre (59.925, -3.7351) radius 1
  circle A294 centre (83.359, 11.27) radius 0.8
  circle A295 centre (75.846, -3.735) radius 0.65
  circle A296 centre (73.306, -3.735) radius 0.65
  circle A297 centre (26.082, 61.562) radius 0.762
  circle A298 centre (85.899, 11.27) radius 0.8
  circle A299 centre (73.3059, -3.7351) radius 1
  circle A300 centre (70.766, -3.735) radius 0.65
  circle A301 centre (30.384, 43.147) radius 0.4
  circle A302 centre (57.3849, -3.735) radius 0.65
  circle A303 centre (26.082, 51.402) radius 0.762
  circle A304 centre (52.498, 31.463) radius 0.762
  circle A305 centre (49.704, 35.654) radius 0.762
  circle A306 centre (47.418, 31.463) radius 0.762
  circle A307 centre (34.6494, 38.194) radius 0.85
  circle A308 centre (65.198, 31.463) radius 0.4572
  circle A309 centre (59.9249, -3.735) radius 0.65
  circle A310 centre (83.359, 11.27) radius 0.5
  circle A311 centre (85.899, 11.27) radius 0.5
  circle A312 centre (62.465, -3.7351) radius 1
  circle A313 centre (26.082, 51.402) radius 0.457
  circle A314 centre (25.508, 9.7549) radius 0.75
  circle A315 centre (28.048, 9.755) radius 0.45
  circle A316 centre (49.0723, 9.7549) radius 0.75
  circle A317 centre (36.2423, -2.1399) radius 1.25
  circle A318 centre (49.0723, 9.755) radius 0.45
  circle A319 centre (30.718, -2.1399) radius 1.25
  circle A320 centre (82.6371, -3.335) radius 1.1
  circle A321 centre (87.6371, -3.335) radius 1.1
  circle A322 centre (36.2423, -2.14) radius 0.8
  circle A323 centre (82.637, -3.335) radius 0.7
  circle A324 centre (20.875, 61.562) radius 0.457
  circle A325 centre (42.7223, 7.2149) radius 0.75
  circle A326 centre (21.698, 7.2149) radius 0.75
  circle A327 centre (26.778, 7.215) radius 0.45
  circle A328 centre (51.7423, -2.14) radius 0.8
  circle A329 centre (45.2623, 7.215) radius 0.45
  circle A330 centre (20.428, 9.755) radius 0.45
  circle A331 centre (30.384, 43.147) radius 0.65
  circle A332 centre (25.508, 9.755) radius 0.45
  circle A333 centre (39.544, 35.654) radius 0.762
  circle A334 centre (26.778, 7.2149) radius 0.75
  circle A335 centre (24.238, 7.215) radius 0.45
  circle A336 centre (15.2179, -2.1399) radius 1.25
  circle A337 centre (20.428, 9.7549) radius 0.75
  circle A338 centre (43.9923, 9.755) radius 0.45
  circle A339 centre (45.2623, 7.2149) radius 0.75
  circle A340 centre (28.384, 43.147) radius 0.4
  circle A341 centre (51.7423, -2.1399) radius 1.25
  circle A342 centre (87.637, -3.335) radius 0.7
  circle A343 centre (28.384, 43.147) radius 0.65
  circle A344 centre (41.4523, 9.755) radius 0.45
  circle A345 centre (30.718, -2.14) radius 0.8
  circle A346 centre (28.048, 9.7549) radius 0.75
  circle A347 centre (43.9923, 9.7549) radius 0.75
  circle A348 centre (46.5323, 9.7549) radius 0.75
  circle A349 centre (49.704, 35.654) radius 0.457
  circle A350 centre (15.218, -2.14) radius 0.8
  circle A351 centre (24.238, 7.2149) radius 0.75
  circle A352 centre (22.968, 9.7549) radius 0.75
  circle A353 centre (47.8023, 7.215) radius 0.45
  circle A354 centre (41.4523, 9.7549) radius 0.75
  circle A355 centre (42.7223, 7.215) radius 0.45
  circle A356 centre (21.698, 7.215) radius 0.45
  circle A357 centre (46.5323, 9.755) radius 0.45
  circle A358 centre (22.968, 9.755) radius 0.45
  circle A359 centre (47.8023, 7.2149) radius 0.75
  circle A360 centre (17.319, 68.2295) radius 1.016
  circle A361 centre (17.253, 0.8649) radius 1.6
  circle A362 centre (86.915, 68.2295) radius 1.016
  circle A363 centre (28.683, 0.8649) radius 1.6
  circle A364 centre (17.319, 33.114) radius 1.016
  circle A365 centre (19.158, 7.2149) radius 0.45
  circle A366 centre (36.623, 16.731) radius 1.016
  circle A367 centre (49.7073, 0.8649) radius 1.6
  circle A368 centre (40.1823, 7.2149) radius 0.45
  circle A369 centre (38.2773, 0.8649) radius 1.6
  circle A370 centre (87.423, 5.555) radius 1.016
  circle A371 centre (80.819, 11.27) radius 0.5
  circle A372 centre (17.319, 68.2295) radius 2.5
  circle A373 centre (86.915, 68.2295) radius 2.5
  circle A374 centre (87.423, 5.555) radius 2.5
  circle A375 centre (36.623, 16.731) radius 2.5
  circle A376 centre (17.319, 33.114) radius 2.5
  point P0 (8, 77)
  point P1 (94.0968, 77)
  point P2 (94.0968, -14.8873)
  point P3 (8, -14)
  dimension "d116" = 5
  dimension "d117" = 5
  dimension "d118" = 5
  dimension "d119" = 5
  dimension "d120" = 5
  constraint concentric A360 A372
  constraint concentric A362 A373
  constraint concentric A370 A374
  constraint concentric A366 A375
  constraint concentric A364 A376
  measures "d116" diameter of A372
  measures "d117" diameter of A373
  measures "d118" diameter of A374
  measures "d119" diameter of A375
  measures "d120" diameter of A376
extrude "Extrude11" add sketch "PCB_Slave_2021-08-24" along normal blind 6 contours A360 | A362 | A364 | A366 | A370 | A372 | A373 | A374 | A375 | A376 bodies 1 in component "Top"
hole "Hole11" at (17.319, 7.5, -93.2295) direction (0, -1, 0) diameter 1.85 depth 5 tip angle 180 bodies 1 in component "Top"
hole "Hole12" at (86.915, 7.5, -93.2295) direction (0, -1, 0) diameter 1.85 depth 5 tip angle 180 bodies 1 in component "Top"
hole "Hole13" at (17.319, 7.5, -58.114) direction (0, -1, 0) diameter 1.85 depth 5 tip angle 180 bodies 1 in component "Top"
hole "Hole14" at (36.623, 7.5, -41.731) direction (0, -1, 0) diameter 1.85 depth 5 tip angle 180 bodies 1 in component "Top"
hole "Hole15" at (87.423, 7.5, -30.555) direction (0, -1, 0) diameter 1.85 depth 5 tip angle 180 bodies 1 in component "Top"
hole "Hole16" at (8, 1.5, -102) at (94.0968, 1.5, -102) at (94.0968, 1.5, -10.1127) at (8, 1.5, -11) direction (0, -1, 0) diameter 3 end through all countersink diameter 6 countersink angle 90 bodies 1 in component "Top"
sketch "Sketch11" plane through (0, 0, 0) normal (0, 0, 1) x (1, 0, 0)
  line L0 (4, 35) -> (4, 0)
  line L1 (4, 0) -> (96, 0)
  line L2 (96, 0) -> (96, 35)
  line L3 (96, 35) -> (4, 35)
  line L4 (37.5432, 17.8974) -> (50.5432, 17.8974)
  line L5 (50.5432, 17.8974) -> (50.5432, 5.8974)
  line L6 (50.5432, 5.8974) -> (37.5432, 5.8974)
  line L7 (37.5432, 5.8974) -> (37.5432, 17.8974)
  circle A0 centre (59.6457, 7.8974) radius 4
  circle A1 centre (84.9963, 7.8974) radius 4
  circle A2 centre (72.3858, 7.8974) radius 4
  dimension "d143" = 13
  dimension "d144" = 12
  dimension "d147" = 8
  dimension "d148" = 8
  dimension "d149" = 8
  constraint horizontal L4
  constraint vertical L5
  constraint horizontal L6
  constraint vertical L7
  measures "d143" distance of L4.start L4.end
  measures "d144" distance of L4.start L6.end
  measures "d147" diameter of A0
  measures "d148" diameter of A1
  measures "d149" diameter of A2
extrude "Extrude12" cut sketch "Sketch11" against normal blind 3 contours L4 L5 L6 L7 | A0 | A1 | A2 bodies 1 in component "Top"
component "Enclosure" placed x (1, 0, 0) y (0, 1, 0) z (0, 0, 1) at (0, 0, 0)
component "Top" placed x (1, 0, 0) y (0, 1, 0) z (0, 0, 1) at (0, 0, 0) in component "Enclosure"
component "Base" placed x (1, 0, 0) y (0, 1, 0) z (0, 0, 1) at (0, 0, 0) in component "Enclosure"
equation "Width = 110 mm"
equation "length = 100 mm"
equation "heigth = 35 mm"
equation "shell = 1.5 mm"
equation "gap = 0.2 mm"
equation "d6 = length"
equation "d7 = Width"
equation "d8 = heigth"
equation "d11 = shell"
equation "d12 = Width / 2"
equation "d13 = shell * 2"
equation "d17 = shell"
equation "d19 = shell + gap"
equation "d20 = shell * 2"
equation "d23 = shell * 2"
equation "d26 = shell"
